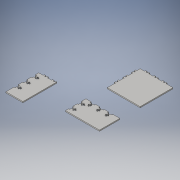
# Autodesk Inventor part: BoxTest
Saved by Autodesk Inventor 2016 (Build 200138000, 138)
## iProperties
Created: 2017-10-17
Part Number: BoxTest
Material: Generic
Document SubType Name: Modeling
Designer: jcj2131
Density: 1 g/cm^3
Appearance: Default
Author: jcj2131
Autodesk Inventor part; units mm, degrees
ref_plane "YZ Plane" through (0, 0, 0) normal (1, 0, 0) x (0, 1, 0)
ref_plane "XZ Plane" through (0, 0, 0) normal (0, 1, 0) x (-1, 0, 0)
ref_plane "XY Plane" through (0, 0, 0) normal (0, 0, 1) x (1, 0, 0)
sketch "Sketch1" plane through (0, 0, 0) normal (0, 1, 0) x (-1, 0, 0)
  line L0 (115.4455, 130) -> (65.4455, 130)
  line L1 (65.4455, 130) -> (65.4455, 30)
  line L2 (65.4455, 30) -> (115.4455, 30)
  line L3 (115.4455, 30) -> (115.4455, 130)
  line L4 (-20.4409, 90) -> (-120.4409, 90)
  line L5 (-120.4409, 90) -> (-120.4409, 30)
  line L6 (-120.4409, 30) -> (-20.4409, 30)
  line L7 (-20.4409, 30) -> (-20.4409, 90)
  line L8 (-20.4409, -30) -> (-120.4409, -30)
  line L9 (-120.4409, -30) -> (-120.4409, -130)
  line L10 (-120.4409, -130) -> (-20.4409, -130)
  line L11 (-20.4409, -130) -> (-20.4409, -30)
  point P0 (0, 0)
  dimension "d0" = 50
  dimension "d1" = 100
  dimension "d2" = 60
  dimension "d3" = 100
  dimension "d4" = 100
  dimension "d5" = 100
  dimension "d8" = 30
  dimension "d9" = 30
  constraints: 24 end point, 6 parallel, 3 horizontal, 3 perpendicular, 2 collinear
  measures "d0" distance of L0.start L0.end
  measures "d1" distance of L2.end L0.start
  measures "d2" distance of L4.end L5.end
  measures "d3" distance of L5.end L6.end
  measures "d4" distance of L10.end L8.start
  measures "d5" distance of L9.end L10.end
  measures "d8" vertical distance of L8.start point (0, 0)
  measures "d9" vertical distance of point (0, 0) L6.end
extrude "Extrusion1" add sketch "Sketch1" along normal blind 3.175
sketch "Sketch2" plane through (0, 3.175, 0) normal (0, 1, 0) x (1, 0, 0)
  line L0 (120.4409, 130) -> (20.4409, 130) projected
  line L1 (20.4409, 130) -> (23.6159, 130)
  line L2 (23.6159, 130) -> (23.6159, 117.3)
  line L3 (23.6159, 117.3) -> (20.4409, 117.3)
  line L4 (20.4409, 117.3) -> (20.4409, 130)
  line L5 (20.4409, 112.7026) -> (23.6159, 112.7026)
  line L6 (23.6159, 112.7026) -> (23.6159, 109.1974)
  line L7 (23.6159, 109.1974) -> (20.4409, 109.1974)
  line L8 (20.4409, 109.1974) -> (20.4409, 112.7026)
  point P0 (0, 0)
  dimension "d10" = 12.7
  dimension "d11" = 3.175
  dimension "d12" = 4.5974
  dimension "d13" = 3.5052
  constraints: 16 end point, 4 parallel, 2 horizontal, 2 perpendicular
  measures "d10" distance of L1.end L2.end
  measures "d11" distance of L2.end L3.end
  measures "d12" distance between parallel lines of L5 L3
  measures "d13" distance of L7.end L5.start
extrude "Extrusion2" cut sketch "Sketch2" against normal through all
pattern_linear "Rectangular Pattern1" count 3 spacing 25.4 along (0, 0, 1) of "Extrusion2"
sketch "Sketch3" plane through (0, 3.175, 0) normal (0, 1, 0) x (1, 0, 0)
  line L0 (120.4409, 130) -> (23.6159, 130) projected
  line L1 (23.6159, 130) -> (36.3159, 130)
  line L2 (36.3159, 130) -> (36.3159, 126.825)
  line L3 (36.3159, 126.825) -> (23.6159, 126.825)
  line L4 (23.6159, 126.825) -> (23.6159, 130)
  line L5 (40.9133, 130) -> (44.4185, 130)
  line L6 (44.4185, 130) -> (44.4185, 126.825)
  line L7 (44.4185, 126.825) -> (40.9133, 126.825)
  line L8 (40.9133, 126.825) -> (40.9133, 130)
  point P0 (0, 0)
  dimension "d19" = 12.7
  dimension "d20" = 3.175
  dimension "d21" = 4.5974
  dimension "d22" = 3.5052
  constraints: 16 end point, 4 parallel, 2 horizontal, 2 perpendicular, 1 point on line
  measures "d19" distance of L2.end L3.end
  measures "d20" distance of L1.end L2.end
  measures "d21" distance between parallel lines of L2 L8
  measures "d22" distance between parallel lines of L6 L8
extrude "Extrusion3" cut sketch "Sketch3" against normal through all
pattern_linear "Rectangular Pattern2" count 3 spacing 25.4 along (1, 0, 0) of "Extrusion3"
sketch "Sketch4" plane through (0, 3.175, 0) normal (0, 1, 0) x (1, 0, 0)
  line L0 (20.4409, 58.3974) -> (20.4409, 30) projected
  line L1 (20.4409, 53.8) -> (23.6159, 53.8)
  line L2 (23.6159, 53.8) -> (23.6159, 30)
  line L3 (23.6159, 30) -> (20.4409, 30)
  line L4 (20.4409, 30) -> (20.4409, 53.8)
  line L5 (23.6159, 58.3974) -> (20.4409, 58.3974) projected
  line L6 (20.4409, 30) -> (120.4409, 30) projected
  point P0 (0, 0)
  dimension "d29" = 3.175
  dimension "d30" = 4.5974
  dimension "d55" = 0
  constraints: 8 end point, 2 parallel, 1 horizontal, 1 perpendicular, 1 point on line
  measures "d29" distance of L2.end L3.end
  measures "d30" distance between parallel lines of L5 L1
  measures "d55" distance between parallel lines of L6 L3
extrude "Extrusion4" cut sketch "Sketch4" against normal through all
sketch "Sketch5" plane through (0, 3.175, 0) normal (0, 1, 0) x (1, 0, 0)
  line L0 (120.4409, 130) -> (95.2185, 130) projected
  line L1 (99.8159, 130) -> (120.4409, 130)
  line L2 (120.4409, 130) -> (120.4409, 126.825)
  line L3 (120.4409, 126.825) -> (99.8159, 126.825)
  line L4 (99.8159, 126.825) -> (99.8159, 130)
  line L5 (95.2185, 130) -> (95.2185, 126.825) projected
  line L6 (120.4409, 30) -> (120.4409, 130) projected
  point P0 (0, 0)
  dimension "d34" = 3.175
  dimension "d35" = 4.5974
  dimension "d73" = 0
  constraints: 8 end point, 2 parallel, 1 horizontal, 1 perpendicular, 1 point on line
  measures "d34" distance of L1.end L2.end
  measures "d35" distance between parallel lines of L5 L4
  measures "d73" distance between parallel lines of L6 L2
extrude "Extrusion5" cut sketch "Sketch5" against normal through all
sketch "Sketch6" plane through (0, 3.175, 0) normal (0, 1, 0) x (1, 0, 0)
  line L0 (-115.4455, -30) -> (-115.4455, -130) projected
  line L1 (-115.4455, -42.7) -> (-112.2705, -42.7)
  line L2 (-112.2705, -42.7) -> (-112.2705, -55.4)
  line L3 (-112.2705, -55.4) -> (-115.4455, -55.4)
  line L4 (-115.4455, -55.4) -> (-115.4455, -42.7)
  line L5 (-65.4455, -30) -> (-115.4455, -30) projected
  line L6 (-112.2705, -47.272) -> (-106.2705, -47.272)
  line L7 (-106.2705, -47.272) -> (-106.2705, -50.828)
  line L8 (-106.2705, -50.828) -> (-112.2705, -50.828)
  line L9 (-112.2705, -50.828) -> (-112.2705, -47.272)
  line L10 (-106.2705, -45.081) -> (-103.4925, -45.081)
  line L11 (-103.4925, -45.081) -> (-103.4925, -53.019)
  line L12 (-103.4925, -53.019) -> (-106.2705, -53.019)
  line L13 (-106.2705, -53.019) -> (-106.2705, -45.081)
  line L14 (-103.4925, -47.272) -> (-100.2055, -47.272)
  line L15 (-100.2055, -47.272) -> (-100.2055, -50.828)
  line L16 (-100.2055, -50.828) -> (-103.4925, -50.828)
  line L17 (-103.4925, -50.828) -> (-103.4925, -47.272)
  point P0 (0, 0)
  dimension "d38" = 12.7
  dimension "d39" = 12.7
  dimension "d40" = 3.175
  dimension "d41" = 6
  dimension "d42" = 4.572
  dimension "d43" = 3.556
  dimension "d44" = 7.938
  dimension "d45" = 2.381
  dimension "d46" = 2.778
  dimension "d47" = 3.287
  dimension "d48" = 3.556
  dimension "d49" = 2.191
  constraints: 32 end point, 8 parallel, 4 horizontal, 4 perpendicular, 4 point on line
  measures "d38" distance between parallel lines of L5 L1
  measures "d39" distance of L1.end L2.end
  measures "d40" distance of L2.end L3.end
  measures "d41" distance of L7.end L8.end
  measures "d42" distance between parallel lines of L1 L6
  measures "d43" distance of L6.end L7.end
  measures "d44" distance of L10.end L11.end
  measures "d45" distance between parallel lines of L1 L10
  measures "d46" distance of L11.end L12.end
  measures "d47" distance of L15.end L16.end
  measures "d48" distance of L14.end L15.end
  measures "d49" distance between parallel lines of L10 L14
extrude "Extrusion6" cut sketch "Sketch6" against normal through all
pattern_linear "Rectangular Pattern3" count 3 spacing 25.4 along (0, 0, 1) of "Extrusion6"
sketch "Sketch7" plane through (0, 3.175, 0) normal (0, 1, 0) x (1, 0, 0)
  line L0 (120.4409, -30) -> (20.4409, -30) projected
  line L1 (36.3159, -30) -> (49.0159, -30)
  line L2 (49.0159, -30) -> (49.0159, -33.175)
  line L3 (49.0159, -33.175) -> (36.3159, -33.175)
  line L4 (36.3159, -33.175) -> (36.3159, -30)
  line L5 (20.4409, -30) -> (20.4409, -90) projected
  line L6 (40.8879, -33.175) -> (44.4439, -33.175)
  line L7 (44.4439, -33.175) -> (44.4439, -39.175)
  line L8 (44.4439, -39.175) -> (40.8879, -39.175)
  line L9 (40.8879, -39.175) -> (40.8879, -33.175)
  line L10 (46.6349, -39.175) -> (38.6969, -39.175)
  line L11 (38.6969, -39.175) -> (38.6969, -41.953)
  line L12 (38.6969, -41.953) -> (46.6349, -41.953)
  line L13 (46.6349, -41.953) -> (46.6349, -39.175)
  line L14 (44.4439, -41.953) -> (40.8879, -41.953)
  line L15 (40.8879, -41.953) -> (40.8879, -45.24)
  line L16 (40.8879, -45.24) -> (44.4439, -45.24)
  line L17 (44.4439, -45.24) -> (44.4439, -41.953)
  point P0 (0, 0)
  dimension "d56" = 15.875
  dimension "d57" = 12.7
  dimension "d58" = 3.175
  dimension "d59" = 6
  dimension "d60" = 3.556
  dimension "d61" = 4.572
  dimension "d62" = 7.938
  dimension "d63" = 2.778
  dimension "d64" = 2.381
  dimension "d65" = 3.287
  dimension "d66" = 3.556
  dimension "d67" = 2.191
  constraints: 32 end point, 8 parallel, 4 horizontal, 4 perpendicular, 4 point on line
  measures "d56" distance between parallel lines of L5 L4
  measures "d57" distance of L2.end L3.end
  measures "d58" distance of L3.end L1.start
  measures "d59" distance of L8.end L6.start
  measures "d60" distance of L7.end L8.end
  measures "d61" distance between parallel lines of L2 L7
  measures "d62" distance of L11.end L12.end
  measures "d63" distance of L10.end L11.end
  measures "d64" distance between parallel lines of L2 L13
  measures "d65" distance of L14.end L15.end
  measures "d66" distance of L15.end L16.end
  measures "d67" distance between parallel lines of L13 L17
extrude "Extrusion7" cut sketch "Sketch7" against normal through all
pattern_linear "Rectangular Pattern4" count 3 spacing 25.4 along (1, 0, 0) of "Extrusion7"
sketch "Sketch8" plane through (0, 3.175, 0) normal (0, 1, 0) x (1, 0, 0)
  line L0 (-65.4455, -30) -> (-115.4455, -30) projected
  line L1 (-115.4455, -30) -> (-102.7455, -30)
  line L2 (-102.7455, -30) -> (-102.7455, -33.175)
  line L3 (-102.7455, -33.175) -> (-115.4455, -33.175)
  line L4 (-115.4455, -33.175) -> (-115.4455, -30)
  line L5 (-98.1485, -30) -> (-94.6435, -30)
  line L6 (-94.6435, -30) -> (-94.6435, -33.175)
  line L7 (-94.6435, -33.175) -> (-98.1485, -33.175)
  line L8 (-98.1485, -33.175) -> (-98.1485, -30)
  point P0 (0, 0)
  dimension "d74" = 3.175
  dimension "d75" = 12.7
  dimension "d76" = 4.597
  dimension "d77" = 3.175
  dimension "d78" = 3.505
  constraints: 16 end point, 4 parallel, 2 horizontal, 2 perpendicular, 1 point on line
  measures "d74" distance of L1.end L2.end
  measures "d75" distance of L2.end L3.end
  measures "d76" distance between parallel lines of L2 L8
  measures "d77" distance of L5.end L6.end
  measures "d78" distance of L6.end L7.end
extrude "Extrusion8" cut sketch "Sketch8" against normal through all
pattern_linear "Rectangular Pattern5" count 2 spacing 25.4 along (1, 0, 0) of "Extrusion8"
sketch "Sketch9" plane through (0, 3.175, 0) normal (0, 1, 0) x (1, 0, 0)
  line L0 (20.4409, -30) -> (20.4409, -90) projected
  line L1 (20.4409, -42.7) -> (23.6159, -42.7)
  line L2 (23.6159, -42.7) -> (23.6159, -55.4)
  line L3 (23.6159, -55.4) -> (20.4409, -55.4)
  line L4 (20.4409, -55.4) -> (20.4409, -42.7)
  line L5 (36.3159, -30) -> (20.4409, -30) projected
  line L6 (23.6159, -47.272) -> (29.6159, -47.272)
  line L7 (29.6159, -47.272) -> (29.6159, -50.828)
  line L8 (29.6159, -50.828) -> (23.6159, -50.828)
  line L9 (23.6159, -50.828) -> (23.6159, -47.272)
  line L10 (29.6159, -45.081) -> (32.3939, -45.081)
  line L11 (32.3939, -45.081) -> (32.3939, -53.019)
  line L12 (32.3939, -53.019) -> (29.6159, -53.019)
  line L13 (29.6159, -53.019) -> (29.6159, -45.081)
  line L14 (32.3939, -47.272) -> (35.6809, -47.272)
  line L15 (35.6809, -47.272) -> (35.6809, -50.828)
  line L16 (35.6809, -50.828) -> (32.3939, -50.828)
  line L17 (32.3939, -50.828) -> (32.3939, -47.272)
  point P0 (0, 0)
  dimension "d84" = 12.7
  dimension "d85" = 12.7
  dimension "d86" = 3.175
  dimension "d87" = 6
  dimension "d88" = 4.572
  dimension "d89" = 3.556
  dimension "d90" = 7.938
  dimension "d91" = 2.381
  dimension "d92" = 2.778
  dimension "d93" = 3.556
  dimension "d94" = 3.287
  dimension "d95" = 2.191
  constraints: 32 end point, 8 parallel, 4 horizontal, 4 perpendicular, 4 point on line
  measures "d84" distance between parallel lines of L5 L1
  measures "d85" distance of L1.end L2.end
  measures "d86" distance of L2.end L3.end
  measures "d87" distance of L7.end L8.end
  measures "d88" distance between parallel lines of L1 L6
  measures "d89" distance of L6.end L7.end
  measures "d90" distance of L10.end L11.end
  measures "d91" distance between parallel lines of L1 L10
  measures "d92" distance of L11.end L12.end
  measures "d93" distance of L14.end L15.end
  measures "d94" distance of L15.end L16.end
  measures "d95" distance between parallel lines of L10 L14
extrude "Extrusion9" cut sketch "Sketch9" against normal through all
pattern_linear "Rectangular Pattern6" count 2 spacing 25.4 along (0, 0, 1) of "Extrusion9"
body "Solid1"
